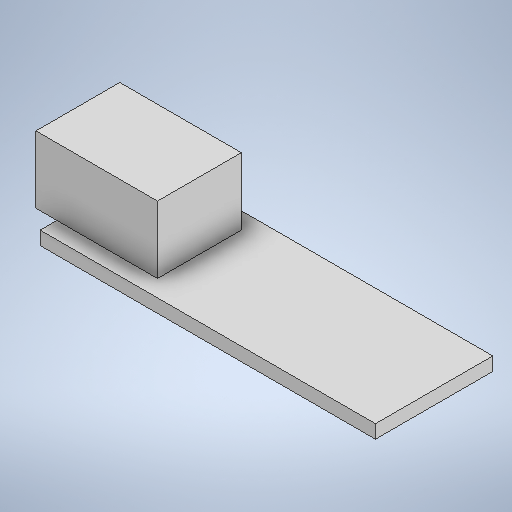
# Autodesk Inventor part: ESP32_PoE
Saved by Autodesk Inventor 2025.2 (Build 292293000, 293)
## iProperties
Created: 2026-03-13
Part Number: ESP32_PoE
Material: Genérico
Document SubType Name: Modeling
Designer: Periscopio
Density: 1 g/cm^3
Appearance: Valor por defecto
Author: Periscopio
Autodesk Inventor part; units mm, degrees
ref_plane "YZ Plane" through (0, 0, 0) normal (1, 0, 0) x (0, 1, 0)
ref_plane "XZ Plane" through (0, 0, 0) normal (0, 1, 0) x (-1, 0, 0)
ref_plane "XY Plane" through (0, 0, 0) normal (0, 0, 1) x (1, 0, 0)
sketch "Boceto1" plane through (0, 0, 0) normal (0, 1, 0) x (-1, 0, 0)
  line L0 (-40, 14) -> (40, 14)
  line L1 (40, 14) -> (40, -14)
  line L2 (40, -14) -> (-40, -14)
  line L3 (-40, -14) -> (-40, 14)
  line L4 (-40, 14) -> (40, -14) construction
  line L5 (40, 14) -> (-40, -14) construction
  point P0 (0, 0)
  dimension "d0" = 80
  dimension "d1" = 28
  constraints: 12 end point, 2 midpoint, 2 parallel, 1 horizontal, 1 perpendicular
  measures "d0" distance of L1.end L2.end
  measures "d1" distance of L0.end L1.end
extrude "Extrusión1" add sketch "Boceto1" along normal blind 3.2
sketch "Boceto2" plane through (0, 3.2, 0) normal (0, 1, 0) x (1, 0, 0)
  line L0 (-45, 10) -> (-16, 10)
  line L1 (-16, 10) -> (-16, -10)
  line L2 (-16, -10) -> (-45, -10)
  line L3 (-45, -10) -> (-45, 10)
  line L4 (-45, 10) -> (-16, -10) construction
  line L5 (-16, 10) -> (-45, -10) construction
  line L6 (-40, 14) -> (-40, -14) projected
  point P0 (0, 0)
  point P1 (-30.5, 0)
  dimension "d4" = 20
  dimension "d5" = 29
  dimension "d6" = 5
  constraints: 12 end point, 2 midpoint, 2 parallel, 1 horizontal, 1 perpendicular
  measures "d4" distance between parallel lines of L2 L0
  measures "d5" distance between parallel lines of L1 L3
  measures "d6" distance between parallel lines of L3 L6
extrude "Extrusión2" add sketch "Boceto2" along normal blind 16
sketch "Boceto3" plane through (-45, 3.2, -10) normal (-1, 0, 0) x (0, 0, 1)
  line L0 (-4, 0) -> (0, 0) projected
  line L1 (20, 0) -> (20, 16) projected
  line L2 (1, 1) -> (19, 1)
  line L3 (19, 1) -> (19, 15)
  line L4 (19, 15) -> (1, 15)
  line L5 (1, 15) -> (1, 1)
  line L6 (1, 1) -> (19, 15) construction
  line L7 (19, 1) -> (1, 15) construction
  point P0 (10, -3.2)
  point P1 (0, 16)
  point P2 (10, 8)
  dimension "d9" = 18
  dimension "d10" = 14
  constraints: 12 end point, 2 midpoint, 2 parallel, 1 horizontal, 1 perpendicular
  measures "d9" distance of L4.end L3.end
  measures "d10" distance of L3.end L2.end
extrude "Extrusión3" cut sketch "Boceto3" against normal blind 10
